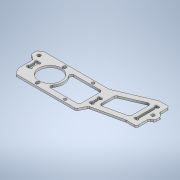
# Autodesk Inventor part: Ankle_side_frame
Saved by Autodesk Inventor 2020.4 (Build 244396000, 396)
## iProperties
Created: 2021-10-01
Part Number: Ankle_side_frame
Material: アルミニウム 2014-T4
Document SubType Name: Modeling
Designer: Masato Kubotera
Density: 2.8 g/cm^3
Appearance: 滑らか - 淡い灰色
Description: A2017 T2
Mass: 9.43206 g
Surface Area: 47.4383 cm^2
Volume: 3.36859 cm^3
Author: Masato Kubotera
Autodesk Inventor part; units mm, degrees
ref_plane "YZ Plane" through (0, 0, 0) normal (1, 0, 0) x (0, 1, 0)
ref_plane "XZ Plane" through (0, 0, 0) normal (0, 1, 0) x (-1, 0, 0)
ref_plane "XY Plane" through (0, 0, 0) normal (0, 0, 1) x (1, 0, 0)
sketch "スケッチ1" plane through (0, 0, 0) normal (0, 0, 1) x (1, 0, 0)
  line L0 (28, 13.5) -> (1, 13.5) construction
  line L1 (1, 13.5) -> (1, -13.5) construction
  line L2 (1, -13.5) -> (28, -13.5) construction
  line L3 (28, -13.5) -> (28, 13.5) construction
  line L4 (28, 13.5) -> (1, -13.5) construction
  line L5 (1, 13.5) -> (28, -13.5) construction
  circle A0 centre (0, 0) radius 10.5 construction
  circle A1 centre (0, 0) radius 10.75
  arc A2 (0, 16) -> (-12, 10.583) centre (0, 0) ccw construction
  line L6 (1, 0) -> (28, 0) construction
  line L7 (14.5, 13.5) -> (14.5, -13.5) construction
  circle A3 centre (28, 13.5) radius 1.35
  arc A4 (-0.35, 12.5) -> (2.35, 12.5) centre (1, 12.5) ccw
  line L8 (2.35, 13.5) -> (2.35, 12.5)
  line L9 (-0.35, 13.5) -> (-0.35, 12.5)
  arc A5 (2.35, 13.5) -> (-0.35, 13.5) centre (1, 13.5) ccw
  line L10 (-12, 10.583) -> (-12, -10.583) construction
  arc A6 (-12, -10.583) -> (0, -16) centre (0, 0) ccw construction
  circle A7 centre (28, -13.5) radius 1.35
  arc A8 (2.35, -12.5) -> (-0.35, -12.5) centre (1, -12.5) ccw
  line L11 (2.35, -13.5) -> (2.35, -12.5)
  line L12 (-0.35, -13.5) -> (-0.35, -12.5)
  arc A9 (-0.35, -13.5) -> (2.35, -13.5) centre (1, -13.5) ccw
  line L13 (-17.5, 5) -> (-14.5, 5) construction
  line L14 (-14.5, 5) -> (-14.5, -5) construction
  line L15 (-14.5, -5) -> (-17.5, -5) construction
  line L16 (-17.5, -5) -> (-17.5, 5) construction
  line L17 (-17.5, 5) -> (-14.5, -5) construction
  line L18 (-14.5, 5) -> (-17.5, -5) construction
  line L19 (-17.51, 5.01) -> (-14.49, 5.01)
  line L20 (-14.49, 5.01) -> (-14.49, 2.91) construction
  line L21 (-14.49, -5.01) -> (-17.51, -5.01)
  line L22 (-17.51, -5.01) -> (-17.51, -2.91) construction
  line L23 (-17.51, 5.01) -> (-14.49, -5.01) construction
  line L24 (-14.49, 5.01) -> (-17.51, -5.01) construction
  arc A10 (-17.51, 5.01) -> (-17.51, 2.91) centre (-17.51, 3.96) ccw
  line L25 (-17.5, 0) -> (-14.5, 0) construction
  line L26 (-16, 5) -> (-16, -5) construction
  arc A11 (-14.49, 2.91) -> (-14.49, 5.01) centre (-14.49, 3.96) ccw
  arc A12 (-17.51, -2.91) -> (-17.51, -5.01) centre (-17.51, -3.96) ccw
  arc A13 (-14.49, -5.01) -> (-14.49, -2.91) centre (-14.49, -3.96) ccw
  line L27 (-17.51, 2.91) -> (-17.51, 5.01) construction
  line L28 (-17.51, -2.91) -> (-17.51, 2.91)
  line L29 (-14.49, -2.91) -> (-14.49, -5.01) construction
  line L30 (-14.49, 2.91) -> (-14.49, -2.91)
  circle A14 centre (-21, 10.5) radius 1.55
  line L31 (-21, 7.0359) -> (-24, 8.7679) construction
  line L32 (-24, 8.7679) -> (-24, 12.2321) construction
  line L33 (-24, 12.2321) -> (-21, 13.9641) construction
  line L34 (-21, 13.9641) -> (-18, 12.2321) construction
  line L35 (-18, 12.2321) -> (-18, 8.7679) construction
  line L36 (-18, 8.7679) -> (-21, 7.0359) construction
  line L37 (-21.4737, 16) -> (-26, 13.3868)
  line L38 (-26, 13.3868) -> (-26, 7.6132)
  line L39 (-26, 7.6132) -> (-20.5, 4.4378)
  line L40 (-20.5, 4.4378) -> (-20.5, -10)
  line L41 (-20.5, -10) -> (-17.0359, -16)
  line L42 (-17.0359, -16) -> (41, -16)
  line L43 (-21.4737, 16) -> (41, 16)
  arc A15 (6.2732, -11.1) -> (6.2732, 11.1) centre (0, 0) ccw
  line L44 (6.2732, 11.1) -> (39, 11.1)
  line L45 (39, 11.1) -> (39, -11.15)
  circle A16 centre (28, 13.5) radius 2.4 construction
  circle A17 centre (28, -13.5) radius 2.4 construction
  line L46 (6.2732, -11.1) -> (39, -11.1)
  line L47 (45, 5) -> (43, 5) construction
  line L48 (43, 5) -> (43, -5) construction
  line L49 (43, -5) -> (45, -5) construction
  line L50 (45, -5) -> (45, 5) construction
  line L51 (45, 5) -> (43, -5) construction
  line L52 (43, 5) -> (45, -5) construction
  line L53 (42.99, 5.01) -> (45.01, 5.01)
  line L54 (45.01, 5.01) -> (45.01, 2.91) construction
  line L55 (45.01, -5.01) -> (42.99, -5.01)
  line L56 (42.99, -5.01) -> (42.99, -2.91) construction
  line L57 (42.99, 5.01) -> (45.01, -5.01) construction
  line L58 (45.01, 5.01) -> (42.99, -5.01) construction
  arc A18 (42.99, 5.01) -> (42.99, 2.91) centre (42.99, 3.96) ccw
  line L59 (43, 0) -> (45, 0) construction
  line L60 (44, 5) -> (44, -5) construction
  arc A19 (45.01, 2.91) -> (45.01, 5.01) centre (45.01, 3.96) ccw
  arc A20 (42.99, -2.91) -> (42.99, -5.01) centre (42.99, -3.96) ccw
  arc A21 (45.01, -5.01) -> (45.01, -2.91) centre (45.01, -3.96) ccw
  line L61 (79.5, 25.4) -> (77.5, 25.4) construction
  line L62 (77.5, 25.4) -> (77.5, 3.6) construction
  line L63 (77.5, 3.6) -> (79.5, 3.6) construction
  line L64 (79.5, 3.6) -> (79.5, 25.4) construction
  line L65 (79.5, 25.4) -> (77.5, 3.6) construction
  line L66 (77.5, 25.4) -> (79.5, 3.6) construction
  line L67 (77.49, 25.41) -> (79.51, 25.41)
  line L68 (79.51, 25.41) -> (79.51, 23.31) construction
  line L69 (79.51, 3.59) -> (77.49, 3.59)
  line L70 (77.49, 3.59) -> (77.49, 5.69) construction
  line L71 (77.49, 25.41) -> (79.51, 3.59) construction
  line L72 (79.51, 25.41) -> (77.49, 3.59) construction
  arc A22 (77.49, 25.41) -> (77.49, 23.31) centre (77.49, 24.36) ccw
  line L73 (78.5, 25.4) -> (78.5, 3.6) construction
  line L74 (77.5, 14.5) -> (79.5, 14.5) construction
  arc A23 (79.51, 23.31) -> (79.51, 25.41) centre (79.51, 24.36) ccw
  arc A24 (77.49, 5.69) -> (77.49, 3.59) centre (77.49, 4.64) ccw
  arc A25 (79.51, 3.59) -> (79.51, 5.69) centre (79.51, 4.64) ccw
  line L75 (42.99, -2.91) -> (42.99, 2.91)
  line L76 (45.01, -2.91) -> (45.01, -5.01) construction
  line L77 (45.01, 2.91) -> (45.01, -2.91)
  line L78 (42.99, 2.91) -> (42.99, 5.01) construction
  line L79 (77.49, 23.31) -> (77.49, 25.41) construction
  line L80 (79.51, 23.31) -> (79.51, 5.69)
  line L81 (79.51, 5.69) -> (79.51, 3.59) construction
  line L82 (77.49, 5.69) -> (77.49, 23.31)
  circle A26 centre (83.5, 15.5) radius 1.55
  line L83 (83.5, 12.0359) -> (80.5, 13.7679) construction
  line L84 (80.5, 13.7679) -> (80.5, 17.2321) construction
  line L85 (80.5, 17.2321) -> (83.5, 18.9641) construction
  line L86 (83.5, 18.9641) -> (86.5, 17.2321) construction
  line L87 (86.5, 17.2321) -> (86.5, 13.7679) construction
  line L88 (86.5, 13.7679) -> (83.5, 12.0359) construction
  line L89 (74.5, 30.4) -> (84.5, 30.4)
  line L90 (84.5, 30.4) -> (84.5, 20.6962)
  line L91 (84.5, 20.6962) -> (88.5, 18.3868)
  line L92 (88.5, 18.3868) -> (88.5, 12.6132)
  line L93 (88.5, 12.6132) -> (84.5, 10.3038)
  line L94 (84.5, 10.3038) -> (84.5, -1.4)
  line L95 (84.5, -1.4) -> (74.5, -1.4)
  line L96 (45, -8) -> (41, -16)
  line L97 (45, -8) -> (74.5, -1.4)
  line L98 (74.5, 30.4) -> (74.5, -1.4) construction
  line L99 (49, 13.9964) -> (49, -1.9815)
  line L100 (49, -1.9815) -> (73.5, 3.4999)
  line L101 (73.5, 3.4999) -> (73.5, 24.5278)
  line L102 (73.5, 24.5278) -> (49, 13.9964)
  line L103 (-17.5, 10) -> (-14.5, 10) construction
  line L104 (-15.0446, -6.3696) -> (-16.9554, -6.3696) construction
  line L105 (-17.5, 10) -> (-15.0446, -6.3696) construction
  line L106 (-14.5, 10) -> (-16.9554, -6.3696) construction
  line L107 (74.5, 30.4) -> (41, 16)
  line L108 (41, 16) -> (41, -16) construction
  point P0 (14.5, 0)
  point P1 (-16, 0)
  point P2 (-16, 0)
  point P3 (44, 0)
  point P4 (44, 0)
  point P5 (78.5, 14.5)
  point P6 (39, -11.1)
  dimension "d0" = 27
  dimension "d1" = 27
  dimension "d2" = 21
  dimension "d3" = 0.25
  dimension "d6" = 2.7
  dimension "d9" = 1
  dimension "d10" = 1.35
  dimension "d11" = 1
  dimension "d12" = 16
  dimension "d13" = 12
  dimension "d14" = 3
  dimension "d16" = 2.5
  dimension "d18" = 0.01
  dimension "d20" = 3.1
  dimension "d21" = 5.5
  dimension "d22" = 6
  dimension "d23" = 0.5
  dimension "d24" = 2
  dimension "d25" = 2
  dimension "d26" = 2
  dimension "d27" = 5
  dimension "d28" = 3
  dimension "d29" = 4.8
  dimension "d52" = 2
  dimension "d53" = 4.8
  dimension "d54" = 10
  dimension "d55" = 0.01
  dimension "d56" = 1.05
  dimension "d66" = 2
  dimension "d67" = 10
  dimension "d68" = 1.05
  dimension "d69" = 0.01
  dimension "d70" = 0.01
  dimension "d71" = 45
  dimension "d72" = 4
  dimension "d75" = 1.05
  dimension "d76" = 0.01
  dimension "d77" = 0.01
  dimension "d78" = 32.5
  dimension "d79" = 14.5
  dimension "d80" = 3.1
  dimension "d86" = 5
  dimension "d87" = 2
  dimension "d88" = 2
  dimension "d89" = 5
  dimension "d90" = 2
  dimension "d91" = 6
  dimension "d92" = 2
  dimension "d93" = 5
  dimension "d94" = 3
  dimension "d95" = 1
  dimension "d96" = 5
  dimension "d97" = 21.8
  dimension "d99" = 3
  dimension "d100" = 2
  dimension "d101" = 4
  dimension "d102" = 4
  dimension "d104" = 5
  dimension "d109" = 5
  dimension "d110" = 5
  constraints: 219 end point, 49 parallel, 38 point on circle, 35 midpoint, 28 symmetric about line, 27 centre point, 19 perpendicular, 17 point on line, 11 horizontal, 10 coincident, 6 tangent, 5 vertical, 1 collinear, 39 other
  measures "d0" distance of L2.end L1.end
  measures "d1" distance of L1.end L0.end
  measures "d2" diameter of A0
  measures "d3" radial gap between concentric circles of A1 A0
  measures "d6" diameter of A3
  measures "d9" distance of A4.centre L0.end
  measures "d10" radius of A5
  measures "d11" distance of point (0, 0) L6.start
  measures "d12" radius of A2
  measures "d13" distance from line of L10 A0.centre
  measures "d14" distance of L14.end L15.end
  measures "d16" distance between parallel lines of L10 L14
  measures "d18" distance between parallel lines of L19 L13
  measures "d20" diameter of A14
  measures "d21" distance from line of L13 A14.centre
  measures "d22" distance between parallel lines of L35 L32
  measures "d23" distance between parallel lines of L16 L35
  measures "d24" distance between parallel lines of L37 L33
  measures "d25" distance between parallel lines of L39 L31
  measures "d26" distance between parallel lines of L38 L32
  measures "d27" distance from line of L40.end L15
  measures "d28" distance between parallel lines of L40 L16
  measures "d29" diameter of A16
  measures "d52" radial gap between concentric circles of A1 A15
  measures "d53" diameter of A17
  measures "d54" distance between parallel lines of L15 L13
  measures "d55" distance between parallel lines of L16 L27
  measures "d56" radius of A10
  measures "d66" distance of L49.end L48.end
  measures "d67" distance of L48.end L47.end
  measures "d68" radius of A18
  measures "d69" distance between parallel lines of L56 L48
  measures "d70" distance between parallel lines of L53 L47
  measures "d71" distance from line of point (0, 0) L50
  measures "d72" distance between parallel lines of L48 L45
  measures "d75" radius of A22
  measures "d76" distance between parallel lines of L61 L67
  measures "d77" distance between parallel lines of L70 L62
  measures "d78" distance between parallel lines of L62 L50
  measures "d79" vertical distance of point (78.5, 14.5) point (44, 0)
  measures "d80" diameter of A26
  measures "d86" distance between parallel lines of L90 L64
  measures "d87" distance between parallel lines of L92 L87
  measures "d88" distance between parallel lines of L91 L86
  measures "d89" horizontal distance of point (83.5, 15.5) point (78.5, 14.5)
  measures "d90" distance between parallel lines of L93 L88
  measures "d91" distance between parallel lines of L88 L85
  measures "d92" distance between parallel lines of L62 L64
  measures "d93" distance between parallel lines of L89 L61
  measures "d94" distance from line of L89.start L62
  measures "d95" vertical distance of point (78.5, 14.5) A26.centre
  measures "d96" distance between parallel lines of L95 L63
  measures "d97" distance between parallel lines of L63 L61
  measures "d99" distance from line of L49 L96.start
  measures "d100" distance from line of L42.end L45
  measures "d101" distance between parallel lines of L50 L99
  measures "d102" distance between parallel lines of L62 L101
  measures "d104" distance between parallel lines of L97 L100
  measures "d109" distance between parallel lines of L13 L103
  measures "d110" distance between parallel lines of L107 L102
extrude "押し出し1" add sketch "スケッチ1" along normal blind 2
fillet "フィレット1" radius 2 17 edges at (-21.4737, 16, 1) (-26, 13.3868, 1) (-26, 7.6132, 1) (-20.5, 4.4378, 1) (-20.5, -10, 1) (-17.0359, -16, 1) (41, 16, 1) (74.5, 30.4, 1) (84.5, 30.4, 1) (84.5, 20.6962, 1) (88.5, 18.3868, 1) (88.5, 12.6132, 1) (84.5, 10.3038, 1) (84.5, -1.4, 1) (74.5, -1.4, 1) (45, -8, 1) (41, -16, 1)
fillet "フィレット2" radius 2 8 edges at (6.2732, 11.1, 1) (6.2732, -11.1, 1) (39, -11.1, 1) (39, 11.1, 1) (49, 13.9964, 1) (49, -1.9815, 1) (73.5, 3.4999, 1) (73.5, 24.5278, 1)
equation "\"d10\" = 0.5 * d6"
equation "\"d25\" = d24"
equation "\"d26\" = d24"
